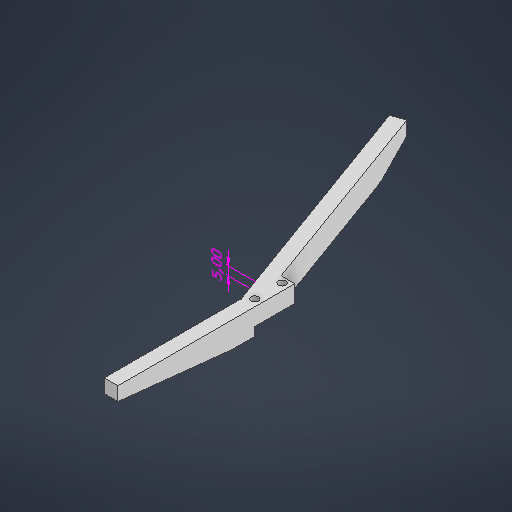
# Autodesk Inventor part: intake arm right
Saved by Autodesk Inventor 2026.1 (Build 301233020, 233B)
## iProperties
Created: 2025-11-05
Part Number: intake arm right
Material: Generic
Document SubType Name: Modeling
Designer: Asus
Density: 1 g/cm^3
Appearance: Default
Author: Asus
Autodesk Inventor part; units mm, degrees
ref_plane "YZ Plane" through (0, 0, 0) normal (1, 0, 0) x (0, 1, 0)
ref_plane "XZ Plane" through (0, 0, 0) normal (0, 1, 0) x (-1, 0, 0)
ref_plane "XY Plane" through (0, 0, 0) normal (0, 0, 1) x (1, 0, 0)
sketch "Sketch1" plane through (0, 0, 0) normal (0, 1, 0) x (-1, 0, 0)
  line L0 (0, 0) -> (8, 0)
  line L1 (8, 0) -> (8, -80)
  line L2 (0, -80) -> (0, 0)
  line L3 (8, -80) -> (57.5929, -216.2554)
  line L4 (8, -80) -> (153, -80) construction
  line L5 (57.5929, -216.2554) -> (50.0754, -218.9916)
  line L6 (50.0754, -218.9916) -> (0.4825, -82.7362)
  line L7 (0.4825, -82.7362) -> (0, -81.4106)
  line L8 (0, -81.4106) -> (0, -80)
  dimension "d3" = 8
  dimension "d4" = 80
  dimension "d6" = 70
  dimension "d7" = 8
  constraints: 18 end point, 3 perpendicular, 2 horizontal, 1 equal length, 1 parallel, 1 vertical
  measures "d3" distance of L1.end L2.start
  measures "d4" distance of L0.end L1.end
  measures "d6" angle of L3 L4
  measures "d7" distance of L3.end L5.end
extrude "Extrusion1" add sketch "Sketch1" along normal blind 8
sketch "Sketch2" plane through (-8, 0, 0) normal (0, 0, 1) x (1, 0, 0)
  line L0 (8, 8) -> (8, 15)
  line L1 (8, 8) -> (0, 8)
  line L2 (8, 8) -> (-42.0754, 8) projected
  line L3 (0, 8) -> (0, 15)
  line L4 (0, 15) -> (8, 15)
  point P0 (8, 0)
  dimension "d10" = 7
  dimension "d11" = 8
  constraints: 8 end point, 2 vertical, 1 perpendicular, 1 point on line
  measures "d10" distance of L0.start L0.end
  measures "d11" distance of L0.start L1.end
extrude "Extrusion2" add sketch "Sketch2" against normal blind 80
sketch "Sketch3" plane through (-57.5929, 0, -216.2554) normal (-0.342, 0, -0.9397) x (-0.9397, 0, 0.342)
  line L0 (-8, 0) -> (-8, 8) projected
  line L1 (0, 0) -> (0, 8) projected
  line L2 (-8, 8) -> (0, 8)
  line L3 (-7.5175, 15) -> (-7.5175, 8) projected
  line L4 (-8, 8) -> (-8, 15)
  line L5 (0, 8) -> (0, 15)
  line L6 (0, 15) -> (-8, 15)
  point P0 (19.8441, 0)
  dimension "d14" = 8
  constraints: 8 end point, 2 vertical, 1 horizontal, 1 perpendicular
  measures "d14" distance of L0.end L1.end
extrude "Extrusion3" add sketch "Sketch3" against normal blind 145
sketch "Sketch8" plane through (0, 0, 0) normal (0, -1, 0) x (1, 0, 0)
  line L0 (-8, -80) -> (-8, 0) projected
  line L1 (-8, -80) -> (0, -80)
  line L2 (0, -80) -> (0, -104)
  line L3 (0, -104) -> (-8, -104)
  line L4 (-8, -104) -> (-8, -80)
  circle A0 centre (-4, -100) radius 2.2
  circle A1 centre (-4, -84) radius 2.2
  point P0 (0, 0)
  point P1 (-4, -80)
  point P2 (-4, -104)
  dimension "d24" = 24
  dimension "d25" = 4.4
  dimension "d26" = 4.4
  dimension "d27" = 4
  dimension "d28" = 4
  constraints: 8 end point, 2 centre point, 2 midpoint, 2 parallel, 1 horizontal, 1 perpendicular
  measures "d24" distance of L1.end L2.end
  measures "d25" diameter of A0
  measures "d26" diameter of A1
  measures "d27" distance of point (-4, -80) A1.centre
  measures "d28" distance of point (-4, -104) A0.centre
extrude "Extrusion7" add sketch "Sketch8" against normal blind 15
sketch "Sketch9" plane through (0, 15, 0) normal (0, 1, 0) x (1, 0, 0)
  line L0 (0, 80) -> (0, 104) projected
  line L1 (-8, 80) -> (-0.4825, 82.7362) projected
  line L2 (0, 104) -> (-8, 104)
  line L3 (-8, 104) -> (-8, 80)
  line L4 (-8, 80) -> (0, 80)
  line L5 (0, 80) -> (0, 104)
  point P0 (0, 0)
  constraints: 8 end point, 2 parallel, 1 horizontal, 1 perpendicular
extrude "Extrusion8" cut sketch "Sketch9" along normal blind 145
extrude "Extrusion9" cut sketch "Sketch8" against normal blind 24 contours A1
sketch "Sketch10" plane through (0, 0, 0) normal (0, -1, 0) x (1, 0, 0)
  line L0 (0, -104) -> (-8, -104) projected
  line L1 (0, 0) -> (0, -104) projected
  line L2 (-8, -104) -> (0, -104)
  line L3 (0, -104) -> (0, -80)
  line L4 (0, -80) -> (-8, -80)
  line L5 (-8, -80) -> (-8, -104)
  dimension "d47" = 24
  constraints: 8 end point, 2 parallel, 1 horizontal, 1 perpendicular, 1 point on line
  measures "d47" distance of L3.end L2.end
extrude "Extrusion10" cut sketch "Sketch10" against normal blind 5
sketch "Sketch11" plane through (0, 5, 0) normal (0, -1, 0) x (1, 0, 0)
  line L0 (0, -104) -> (-8, -104) projected
  line L1 (-50.0754, -218.9916) -> (-8, -103.3904) projected
  line L2 (0, -104) -> (-8, -104)
  line L3 (-8, -104) -> (-8, -103.3904)
  line L4 (-8, -103.3904) -> (0, -103.3904)
  line L5 (0, -103.3904) -> (0, -104)
  point P0 (0, 0)
  constraints: 8 end point, 2 parallel, 1 horizontal, 1 perpendicular
extrude "Extrusion11" cut sketch "Sketch11" against normal blind 13
chamfer "Chamfer3" distance 7 angle 84 1 edges at (-4, 0, 0) measured on face at (-5.3333, 5, 0)
chamfer "Chamfer4" distance 7 angle 75 1 edges at (-53.8342, 0, -217.6235) measured on face at (-55.0871, 5, -217.1675)
body "Solid1"
